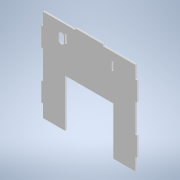
# Autodesk Inventor part: Suelo
Saved by Autodesk Inventor 2020.1 (Build 241239000, 239)
## iProperties
Created: 2019-12-08
Part Number: Suelo
Material: Generic
Document SubType Name: Modeling
Designer: Daniel
Density: 1 g/cm^3
Appearance: Default
Author: Daniel
Autodesk Inventor part; units mm, degrees
ref_plane "YZ Plane" through (0, 0, 0) normal (1, 0, 0) x (0, 1, 0)
ref_plane "XZ Plane" through (0, 0, 0) normal (0, 1, 0) x (-1, 0, 0)
ref_plane "XY Plane" through (0, 0, 0) normal (0, 0, 1) x (1, 0, 0)
sketch "Sketch1" plane through (0, 0, 0) normal (1, 0, 0) x (0, 1, 0)
  line L0 (-40.5, -1.5) -> (40.5, -1.5)
  line L1 (40.5, -1.5) -> (40.5, 1.5)
  line L2 (40.5, 1.5) -> (-40.5, 1.5)
  line L3 (-40.5, 1.5) -> (-40.5, -1.5)
  line L4 (-40.5, -1.5) -> (40.5, 1.5) construction
  line L5 (40.5, -1.5) -> (-40.5, 1.5) construction
  point P0 (0, 0)
  point P1 (0, 0)
  point P2 (0, 0)
  dimension "d27" = 3
  dimension "d28" = 81
  constraints: 12 end point, 3 midpoint, 2 parallel, 1 coincident, 1 horizontal, 1 perpendicular, 1 other
  measures "d27" distance of L0.end L1.end
  measures "d28" distance of L1.end L2.end
extrude "Extrusion1" add sketch "Sketch1" along normal mid plane 88
sketch "Sketch2" plane through (44, 0, 0) normal (1, 0, 0) x (0, 0, -1)
  line L0 (1.5, 40.5) -> (-1.5, 40.5) projected
  line L1 (-1.5, 40.5) -> (-1.5, -40.5) projected
  line L2 (-1.5, -40.5) -> (1.5, -40.5) projected
  line L3 (1.5, -40.5) -> (1.5, 40.5) projected
  line L4 (1.5, 40.5) -> (-1.5, 40.5)
  line L5 (-1.5, 40.5) -> (-1.5, -127.5)
  line L6 (-1.5, -127.5) -> (1.5, -127.5)
  line L7 (1.5, -127.5) -> (1.5, 40.5)
  line L8 (-1.5, 40.5) -> (-1.5, -40.5) projected
  point P0 (0, 0)
  dimension "d29" = 168
  constraints: 8 end point, 2 parallel, 1 collinear, 1 horizontal, 1 perpendicular
  measures "d29" distance between parallel lines of L0 L6
extrude "Extrusion2" add sketch "Sketch2" along normal blind 40
sketch "Sketch3" plane through (44, -35, 1.5) normal (0, 0, 1) x (1, 0, 0)
  line L0 (-44, 35) -> (111.2969, 35) construction
  line L1 (43, 17.5) -> (40, 17.5)
  line L2 (40, 17.5) -> (40, 52.5)
  line L3 (40, 52.5) -> (43, 52.5)
  line L4 (43, 52.5) -> (43, 17.5)
  line L5 (43, 17.5) -> (40, 52.5) construction
  line L6 (40, 17.5) -> (43, 52.5) construction
  line L7 (40, 75.5) -> (40, -92.5) projected
  line L8 (0, -5.5) -> (0, -92.5) projected
  line L9 (0, -92.5) -> (40, -92.5) projected
  line L10 (40, -92.5) -> (40, 75.5) projected
  line L11 (40, -8.5) -> (0, -8.5) construction
  line L12 (43, -34.5) -> (40, -34.5)
  line L13 (40, -34.5) -> (40, -69.5)
  line L14 (40, -69.5) -> (43, -69.5)
  line L15 (43, -69.5) -> (43, -34.5)
  line L16 (43, -34.5) -> (40, -69.5) construction
  line L17 (40, -34.5) -> (43, -69.5) construction
  point P0 (41.5, 35)
  point P1 (41.5, -52)
  point P2 (40, -34.5)
  point P3 (40, -69.5)
  dimension "d23" = 3
  dimension "d24" = 35
  constraints: 28 end point, 5 midpoint, 5 symmetric about line, 2 horizontal, 2 parallel, 2 perpendicular, 2 point on line, 1 collinear, 1 other
  measures "d23" distance of L2.end L3.end
  measures "d24" distance of L3.end L1.start
extrude "Extrusion3" add sketch "Sketch3" against normal up to surface (3 mm away)
mirror "Mirror1" about plane through (0, 0, 0) normal (1, 0, 0) of "Extrusion2", "Extrusion3"
sketch "Sketch4" plane through (84, -127.5, -1.5) normal (0, 0, -1) x (-1, 0, 0)
  line L0 (40, 153) -> (43, 153)
  line L1 (43, 153) -> (43, 138)
  line L2 (43, 138) -> (40, 138)
  line L3 (40, 138) -> (40, 153)
  line L4 (40, 20) -> (43, 20)
  line L5 (43, 55) -> (43, 20)
  line L6 (43, 82.6608) -> (43, 55)
  line L7 (40, 82.6608) -> (43, 82.6608)
  line L8 (40, 55) -> (40, 82.6608)
  line L9 (43, 55) -> (40, 55)
  line L10 (40, 20) -> (40, 55)
  line L11 (40, -14.5469) -> (40, 20)
  line L12 (43, -14.5469) -> (40, -14.5469)
  line L13 (43, 20) -> (43, -14.5469)
  line L14 (125, 153) -> (128, 153)
  line L15 (128, 153) -> (128, 138)
  line L16 (128, 138) -> (125, 138)
  line L17 (125, 138) -> (125, 153)
  line L18 (125, 20) -> (128, 20)
  line L19 (128, 55) -> (128, 20)
  line L20 (128, 82.6608) -> (128, 55)
  line L21 (125, 82.6608) -> (128, 82.6608)
  line L22 (125, 55) -> (125, 82.6608)
  line L23 (128, 55) -> (125, 55)
  line L24 (125, 20) -> (125, 55)
  line L25 (125, -14.5469) -> (125, 20)
  line L26 (128, -14.5469) -> (125, -14.5469)
  line L27 (128, 20) -> (128, -14.5469)
  point P0 (84, 127.5)
  constraints: 56 end point, 16 vertical, 12 horizontal, 24 other
extrude "Extrusion4" cut sketch "Sketch4" against normal blind 10 contours L0 L1 L2 L3 | L14 L15 L16 L17
sketch "Sketch5" plane through (44, -127.5, -1.5) normal (0, 0, -1) x (-1, 0, 0)
  line L0 (99.9, 138) -> (99.9, 147)
  line L1 (89.6, 147) -> (89.6, 138)
  line L2 (89.6, 138) -> (99.9, 138)
  line L3 (94.75, 147) -> (94.75, 138) construction
  line L4 (89.75, 147) -> (89.75, 138)
  line L5 (99.75, 138) -> (99.75, 147)
  arc A0 (99.75, 147) -> (89.75, 147) centre (94.75, 147) ccw
  arc A1 (89.75, 138) -> (99.75, 138) centre (94.75, 138) ccw
  point P0 (44, 127.5)
  point P1 (94.75, 142.5)
  dimension "d35" = 10
  dimension "d36" = 9
  dimension "d37" = 0.15
  dimension "d38" = 55.9
  dimension "d39" = 10.5
  dimension "d40" = 9
  dimension "d41" = 9
  constraints: 14 end point, 4 point on circle, 4 tangent, 3 parallel, 2 centre point, 2 midpoint, 1 horizontal, 1 vertical
  measures "d35" diameter of A1
  measures "d36" distance from line of L5.end L2
  measures "d37" distance between parallel lines of L0 L5
  measures "d38" distance from line of point (44, 127.5) L0
  measures "d39" distance from line of point (44, 127.5) L2
  measures "d40" distance from line of L0.end L2
  measures "d41" distance from line of L1.start L2
extrude "Extrusion5" cut sketch "Sketch5" against normal blind 10
sketch "Sketch6" plane through (44, -127.5, 1.5) normal (0, 0, 1) x (1, 0, 0)
  line L0 (-69, 165) -> (-19, 165)
  line L1 (-19, 165) -> (-19, 171)
  line L2 (-19, 171) -> (-69, 171)
  line L3 (-69, 171) -> (-69, 165)
  line L4 (40, 168) -> (-128, 168) projected
  line L5 (-69, 165) -> (-19, 171) construction
  line L6 (-19, 165) -> (-69, 171) construction
  point P0 (-44, 127.5)
  point P1 (-44, 168)
  point P2 (-69, 168)
  point P3 (-19, 168)
  dimension "d44" = 50
  dimension "d45" = 6
  constraints: 12 end point, 3 midpoint, 2 parallel, 1 horizontal, 1 perpendicular
  measures "d44" distance of L1.end L2.end
  measures "d45" distance of L0.end L1.end
extrude "Extrusion6" add sketch "Sketch6" against normal up to surface (3 mm away) contours L3 L2 L1 L4
body "Solid1"
